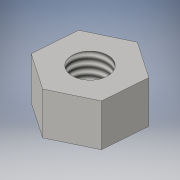
# Autodesk Inventor part: Threaded Rod Nut
Saved by Autodesk Inventor 2016 (Build 200138000, 138)
## iProperties
Created: 2016-04-14
Part Number: Threaded Rod Nut
Material: Aluminum 6061
Document SubType Name: Modeling
Designer: rmarkowi
Density: 2.7 g/cm^3
Appearance: Aluminum - Flat
Author: rmarkowi
Autodesk Inventor part; units mm, degrees
ref_plane "YZ Plane" through (0, 0, 0) normal (1, 0, 0) x (0, 1, 0)
ref_plane "XZ Plane" through (0, 0, 0) normal (0, 1, 0) x (-1, 0, 0)
ref_plane "XY Plane" through (0, 0, 0) normal (0, 0, 1) x (1, 0, 0)
sketch "Sketch1" plane through (0, 0, 0) normal (0, 1, 0) x (-1, 0, 0)
  line L0 (10.5852, -7.2528) -> (-0.9885, -12.7935)
  line L1 (-0.9885, -12.7935) -> (-11.5737, -5.5406)
  line L2 (-11.5737, -5.5406) -> (-10.5852, 7.2528)
  line L3 (-10.5852, 7.2528) -> (0.9885, 12.7935)
  line L4 (0.9885, 12.7935) -> (11.5737, 5.5406)
  line L5 (11.5737, 5.5406) -> (10.5852, -7.2528)
  point P0 (0, 0)
  point P1 (0, 0)
  dimension "d0" = 22.225
  constraints: 12 end point, 1 coincident, 13 other
  measures "d0" distance between parallel lines of L1 L4
extrude "Extrusion1" add sketch "Sketch1" along normal blind 12.3031
sketch "Sketch2" plane through (0, 12.3031, 0) normal (0, 1, 0) x (1, 0, 0)
  line L0 (-10.5852, 7.2528) -> (-11.5737, -5.5406) construction
  line L1 (11.5737, 5.5406) -> (0.9885, 12.7935) construction
  line L2 (-11.5737, -5.5406) -> (11.5737, 5.5406) construction
  line L3 (10.5852, -7.2528) -> (11.5737, 5.5406) construction
  line L4 (11.5737, 5.5406) -> (10.5852, -7.2528) construction
  line L5 (0.9885, 12.7935) -> (-10.5852, 7.2528) construction
  line L6 (10.5852, -7.2528) -> (-10.5852, 7.2528) construction
  point P0 (0, 0)
  constraints: 6 end point, 1 collinear, 1 parallel
hole "Hole1" at (0, 12.3031, 0) direction (0, -1, 0) diameter 10.414 end through all thread size "1/2-12 UNS" class "2B" standard "ANSI Unified Screw Threads"
body "Solid1"
